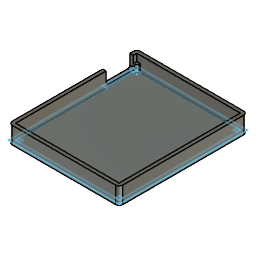
radpad_bottom (Autodesk Fusion 360 design; units mm, degrees)
part number: 2026-05-31-12-24-51-913
Autodesk Fusion 360 part; units mm, degrees
sketch "Sketch1" plane through (0, 0, 0) normal (0, 0, 1) x (1, 0, 0)
  line L0 (-21, 20) -> (67.2, 20)
  line L1 (67.2, 20) -> (67.2, -83.2)
  line L2 (67.2, -83.2) -> (-21, -83.2)
  line L3 (-21, -83.2) -> (-21, 20)
  line L4 (-24, 23) -> (70.2, 23)
  line L5 (70.2, 23) -> (70.2, -86.2)
  line L6 (70.2, -86.2) -> (-24, -86.2)
  line L7 (-24, -86.2) -> (-24, 23)
  line L8 (-21, 20) -> (-24, 20)
  line L9 (-24, 20) -> (-24, -6.1)
  line L10 (-24, -6.1) -> (-21, -6.1)
  line L11 (-21, -6.1) -> (-21, 20)
  line L12 (-21, 20) -> (-18, 20)
  line L13 (-18, 20) -> (-18, 17)
  line L14 (-18, 17) -> (-21, 17)
  line L15 (-21, 17) -> (-21, 20)
  line L16 (67.2, 20) -> (64.2, 20)
  line L17 (64.2, 20) -> (64.2, 17)
  line L18 (64.2, 17) -> (67.2, 17)
  line L19 (67.2, 17) -> (67.2, 20)
  line L20 (-21, -83.2) -> (-18, -83.2)
  line L21 (-18, -83.2) -> (-18, -80.2)
  line L22 (-18, -80.2) -> (-21, -80.2)
  line L23 (-21, -80.2) -> (-21, -83.2)
  line L24 (67.2, -83.2) -> (64.2, -83.2)
  line L25 (64.2, -83.2) -> (64.2, -80.2)
  line L26 (64.2, -80.2) -> (67.2, -80.2)
  line L27 (67.2, -80.2) -> (67.2, -83.2)
  line L28 (-24, 20) -> (-21, 20)
  line L29 (-21, 20) -> (-21, 17)
  line L30 (-21, 17) -> (-24, 17)
  line L31 (-24, 17) -> (-24, 20)
  dimension "d1" = 88.2
  dimension "d2" = 103.2
  dimension "d3" = 94.2
  dimension "d4" = 109.2
  dimension "d5" = 3
  dimension "d6" = 3
  dimension "d7" = 3
  dimension "d8" = 26.1
  dimension "d9" = 3
  dimension "d10" = 3
  dimension "d11" = 3
  dimension "d12" = 3
  dimension "d13" = 3
  dimension "d14" = 3
  dimension "d15" = 3
  dimension "d16" = 3
  constraint horizontal L0
  constraint vertical L1
  constraint horizontal L2
  constraint vertical L3
  constraint horizontal L4
  constraint vertical L5
  constraint horizontal L6
  constraint vertical L7
  constraint horizontal L8
  constraint vertical L9
  constraint horizontal L10
  constraint vertical L11
  constraint horizontal L12
  constraint vertical L13
  constraint horizontal L14
  constraint vertical L15
  constraint horizontal L16
  constraint vertical L17
  constraint horizontal L18
  constraint vertical L19
  constraint horizontal L20
  constraint vertical L21
  constraint horizontal L22
  constraint vertical L23
  constraint horizontal L24
  constraint vertical L25
  constraint horizontal L26
  constraint vertical L27
  constraint horizontal L28
  constraint vertical L29
  constraint horizontal L30
  constraint vertical L31
  measures "d1" distance of L0.start L0.end
  measures "d2" distance of L0.start L2.end
  measures "d3" distance of L4.start L4.end
  measures "d4" distance of L4.start L6.end
  measures "d5" distance of L0 L4
  measures "d6" distance of L3 L7
  measures "d7" distance of L0.start L8.end
  measures "d8" distance of L0.start L10.end
  measures "d9" distance of L0.start L12.end
  measures "d10" distance of L0.start L14.end
  measures "d11" distance of L0.end L16.end
  measures "d12" distance of L0.end L18.end
  measures "d13" distance of L2.end L20.end
  measures "d14" distance of L2.end L22.end
  measures "d15" distance of L1.end L24.end
  measures "d16" distance of L1.end L26.end
extrude "Extrude1" add sketch "Sketch1" against normal blind 2 makes body 1
extrude "Extrude2" add sketch "Sketch1" along normal blind 6.4 separate body contours L0 L3 L11 L12 L13 L14 L15 L29 | L0 L1 L16 L17 L18 L19 | L2 L3 L20 L21 L22 L23 | L1 L2 L24 L25 L26 L27 makes body 2 at (65.2, 20, 2.1333) makes body 3 at (-18, -82.2, 2.1333) makes body 4 at (-20, 20, 2.1333) makes body 5 at (67.2, -81.2, 2.1333)
extrude "Extrude3" add sketch "Sketch1" along normal blind 12.5 contours L0 L1 L2 L3 L4 L5 L6 L7 L8 L10 L12 L16 L19 L20 L23 L24 L27 L28 bodies 1 2 3 4 5
extrude "Extrude4" add sketch "Sketch1" along normal blind 12.5 separate body contours L3 L7 L8 L9 L11 L15 L28 L29 L30 L31 makes body 6
fillet "Fillet1" radius 3 4 edges at (-24, -86.2, 5.25) (70.2, -86.2, 5.25) (70.2, 23, 5.25) (-24, 23, 5.25) on bodies 1
fillet "Fillet2" radius 2 1 edges at (-18, 17, 3.2) on bodies 1
fillet "Fillet3" radius 2 3 edges at (64.2, 17, 3.2) (64.2, -80.2, 3.2) (-18, -80.2, 3.2) on bodies 1
extrude "Extrude5" add sketch "Sketch1" along normal blind 2 contours L3 L7 L9 L10 L11 L30 bodies 1 6
fillet "Fillet4" radius 2 2 edges at (-22.5, 17, 2) (-22.5, -6.1, 2) on bodies 1
